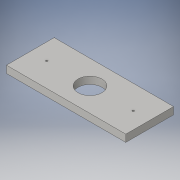
# Autodesk Inventor part: Pimount
Saved by Autodesk Inventor 2016 (Build 200138000, 138)
## iProperties
Created: 2016-02-22
Part Number: Pimount
Material: Generic
Document SubType Name: Modeling
Designer: Scott
Density: 1 g/cm^3
Appearance: Default
Author: Scott
Autodesk Inventor part; units mm, degrees
ref_plane "YZ Plane" through (0, 0, 0) normal (1, 0, 0) x (0, 1, 0)
ref_plane "XZ Plane" through (0, 0, 0) normal (0, 1, 0) x (-1, 0, 0)
ref_plane "XY Plane" through (0, 0, 0) normal (0, 0, 1) x (1, 0, 0)
sketch "Sketch1" plane through (0, 0, 0) normal (0, 1, 0) x (-1, 0, 0)
  line L0 (0, 0) -> (63.5, 0)
  line L1 (63.5, 0) -> (63.5, -25.4)
  line L2 (63.5, -25.4) -> (0, -25.4)
  line L3 (0, -25.4) -> (0, 0)
  dimension "d0" = 63.5
  dimension "d1" = 25.4
  constraints: 8 end point, 2 parallel, 1 horizontal, 1 perpendicular
  measures "d0" distance of L1.end L2.end
  measures "d1" distance of L0.end L1.end
extrude "Extrusion1" add sketch "Sketch1" along normal blind 3.81
sketch "Sketch2" plane through (0, 3.81, 0) normal (0, 1, 0) x (1, 0, 0)
  line L0 (-63.5, 0) -> (0, 0) projected
  line L1 (0, 0) -> (0, 25.4) projected
  line L2 (0, 25.4) -> (-63.5, 25.4) projected
  line L3 (-63.5, 25.4) -> (-63.5, 0) projected
  line L4 (-31.75, 12.7) -> (-54.75, 12.7)
  line L5 (-31.75, 12.7) -> (-8.75, 12.7)
  circle A0 centre (-54.75, 12.7) radius 0.5
  circle A1 centre (-8.75, 12.7) radius 0.5
  circle A2 centre (-31.75, 12.7) radius 6.35
  dimension "d4" = 23
  dimension "d5" = 23
  dimension "d6" = 1
  dimension "d7" = 1
  dimension "d8" = 12.7
  constraints: 4 end point, 3 centre point, 3 coincident, 2 horizontal
  measures "d4" distance of L4.start L4.end
  measures "d5" distance of L4.start L5.end
  measures "d6" diameter of A0
  measures "d7" diameter of A1
  measures "d8" diameter of A2
extrude "Extrusion2" cut sketch "Sketch2" against normal blind 3.81 contours L5 A2 L4 | L4 A2 L5 | A0 | A1
body "Solid1"
